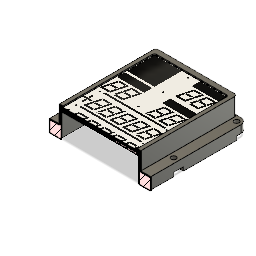
DSKY front frame mechanical 3D (Autodesk Fusion 360 design; units mm, degrees)
Autodesk Fusion 360 part; units mm, degrees
sketch "Sketch1" plane through (0, 0, 0) normal (0, 1, 0) x (1, 0, 0)
  line L0 (-36.322, 56.134) -> (36.322, 56.134)
  line L1 (41.402, 51.054) -> (41.402, -51.054)
  line L2 (36.322, -56.134) -> (-36.322, -56.134)
  line L3 (-41.402, -51.054) -> (-41.402, 51.054)
  line L4 (-41.402, 56.134) -> (41.402, -56.134) construction
  line L5 (41.402, 56.134) -> (-41.402, -56.134) construction
  arc A0 (-36.322, 56.134) -> (-41.402, 51.054) centre (-36.322, 51.054) ccw
  arc A1 (41.402, 51.054) -> (36.322, 56.134) centre (36.322, 51.054) ccw
  arc A2 (36.322, -56.134) -> (41.402, -51.054) centre (36.322, -51.054) ccw
  arc A3 (-41.402, -51.054) -> (-36.322, -56.134) centre (-36.322, -51.054) ccw
  line L6 (-30.988, 56.134) -> (30.988, 56.134)
  line L7 (33.274, 53.848) -> (33.274, -53.848)
  line L8 (30.988, -56.134) -> (-30.988, -56.134)
  line L9 (-33.274, -53.848) -> (-33.274, 53.848)
  line L10 (-33.274, 56.134) -> (33.274, -56.134) construction
  line L11 (33.274, 56.134) -> (-33.274, -56.134) construction
  arc A4 (-30.988, 56.134) -> (-33.274, 53.848) centre (-30.988, 53.848) ccw
  arc A5 (33.274, 53.848) -> (30.988, 56.134) centre (30.988, 53.848) ccw
  arc A6 (30.988, -56.134) -> (33.274, -53.848) centre (30.988, -53.848) ccw
  arc A7 (-33.274, -53.848) -> (-30.988, -56.134) centre (-30.988, -53.848) ccw
  line L12 (-28.702, 51.8795) -> (28.702, 51.8795)
  line L13 (30.226, 50.3555) -> (30.226, -50.3555)
  line L14 (28.702, -51.8795) -> (-28.702, -51.8795)
  line L15 (-30.226, -50.3555) -> (-30.226, 50.3555)
  line L16 (-30.226, 51.8795) -> (30.226, -51.8795) construction
  line L17 (30.226, 51.8795) -> (-30.226, -51.8795) construction
  arc A8 (-28.702, 51.8795) -> (-30.226, 50.3555) centre (-28.702, 50.3555) ccw
  arc A9 (30.226, 50.3555) -> (28.702, 51.8795) centre (28.702, 50.3555) ccw
  arc A10 (28.702, -51.8795) -> (30.226, -50.3555) centre (28.702, -50.3555) ccw
  arc A11 (-30.226, -50.3555) -> (-28.702, -51.8795) centre (-28.702, -50.3555) ccw
  line L18 (-30.456, 53.3795) -> (30.456, 53.3795)
  line L19 (31.726, 52.1095) -> (31.726, -52.1095)
  line L20 (30.456, -53.3795) -> (-30.456, -53.3795)
  line L21 (-31.726, -52.1095) -> (-31.726, 52.1095)
  line L22 (-31.726, 53.3795) -> (31.726, -53.3795) construction
  line L23 (31.726, 53.3795) -> (-31.726, -53.3795) construction
  arc A12 (-30.456, 53.3795) -> (-31.726, 52.1095) centre (-30.456, 52.1095) ccw
  arc A13 (31.726, 52.1095) -> (30.456, 53.3795) centre (30.456, 52.1095) ccw
  arc A14 (30.456, -53.3795) -> (31.726, -52.1095) centre (30.456, -52.1095) ccw
  arc A15 (-31.726, -52.1095) -> (-30.456, -53.3795) centre (-30.456, -52.1095) ccw
  line L24 (37.338, 51.562) -> (-37.338, 51.562) construction
  line L25 (-37.338, 51.562) -> (-37.338, -51.562) construction
  line L26 (-37.338, -51.562) -> (37.338, -51.562) construction
  line L27 (37.338, -51.562) -> (37.338, 51.562) construction
  line L28 (37.338, 51.562) -> (-37.338, -51.562) construction
  line L29 (-37.338, 51.562) -> (37.338, -51.562) construction
  circle A16 centre (-37.338, 51.562) radius 2.032
  circle A17 centre (37.338, 51.562) radius 2.032
  circle A18 centre (37.338, 0) radius 2.032
  circle A19 centre (37.338, -51.562) radius 2.032
  circle A20 centre (-37.338, -51.562) radius 2.032
  circle A21 centre (-37.338, 0) radius 2.032
  dimension "d1" = 82.804
  dimension "d2" = 112.268
  dimension "d3" = 5.08
  dimension "d4" = 66.548
  dimension "d5" = 2.286
  dimension "d6" = 60.452
  dimension "d7" = 103.759
  dimension "d8" = 1.524
  dimension "d15" = 1.5
  dimension "d16" = 1.5
  dimension "d17" = 1.27
  dimension "d21" = 4.064
  dimension "d22" = 74.676
  dimension "d23" = 103.124
  measures "d3" radius of A0
  measures "d4" distance of L7 L9
  measures "d5" radius of A4
  measures "d8" radius of A8
  measures "d15" distance of L12 L18
  measures "d16" distance of L15 L21
  measures "d17" radius of A12
  measures "d21" diameter of A17
  measures "d22" distance of L25 L27
  measures "d23" distance of L24 L26
extrude "Extrude1" add sketch "Sketch1" against normal blind 23.876 contours L0 L2 L3 A0 A3 L9 A4 A7 | L0 L2 L6 L7 L8 L9 A4 A5 A6 A7 | L0 L1 L2 A1 A2 L7 A5 A6 | L12 L13 L14 L15 A8 A9 A10 A11 | L18 L19 L20 L21 A12 A13 A14 A15 | A16 | A17 | A18 | A19 | A20 | A21 makes body 1
extrude "Extrude2" cut sketch "Sketch1" against normal blind 14.351 contours L0 L2 L3 A0 A3 L9 A4 A7 | L0 L1 L2 A1 A2 L7 A5 A6 | A16 | A17 | A18 | A19 | A20 | A21 bodies 1
extrude "Extrude3" cut sketch "Sketch1" against normal blind 70 contours L12 L13 L14 L15 A8 A9 A10 A11 bodies 1
extrude "Extrude4" cut sketch "Sketch1" against normal blind 40 from surface at -1 contours L18 L19 L20 L21 A12 A13 A14 A15 bodies 1
extrude "Extrude5" cut sketch "Sketch1" against normal blind 80 contours A16 | A17 | A18 | A19 | A20 | A21 bodies 1
sketch "Sketch2" plane through (0, -23.876, 0) normal (0, -1, 0) x (1, 0, 0)
  circle A0 centre (37.338, 51.562) radius 2.032
  circle A1 centre (-37.338, -51.562) radius 2.032
  circle A2 centre (37.338, 0) radius 2.032
  circle A3 centre (-37.338, 51.562) radius 2.032
  circle A4 centre (-37.338, 0) radius 2.032
  circle A5 centre (37.338, -51.562) radius 2.032
  line L0 (-31.726, -52.1095) -> (-31.726, 52.1095)
  arc A6 (-30.456, 53.3795) -> (-31.726, 52.1095) centre (-30.456, 52.1095) ccw
  line L1 (-30.456, 53.3795) -> (30.456, 53.3795)
  arc A7 (31.726, 52.1095) -> (30.456, 53.3795) centre (30.456, 52.1095) ccw
  line L2 (31.726, 52.1095) -> (31.726, -52.1095)
  arc A8 (30.456, -53.3795) -> (31.726, -52.1095) centre (30.456, -52.1095) ccw
  line L3 (30.456, -53.3795) -> (-30.456, -53.3795)
  arc A9 (-31.726, -52.1095) -> (-30.456, -53.3795) centre (-30.456, -52.1095) ccw
  arc A10 (41.402, 51.054) -> (36.322, 56.134) centre (36.322, 51.054) ccw
  line L4 (36.322, 56.134) -> (-36.322, 56.134)
  arc A11 (-36.322, 56.134) -> (-41.402, 51.054) centre (-36.322, 51.054) ccw
  line L5 (-41.402, 51.054) -> (-41.402, -51.054)
  arc A12 (-41.402, -51.054) -> (-36.322, -56.134) centre (-36.322, -51.054) ccw
  line L6 (-36.322, -56.134) -> (36.322, -56.134)
  arc A13 (36.322, -56.134) -> (41.402, -51.054) centre (36.322, -51.054) ccw
  line L7 (41.402, -51.054) -> (41.402, 51.054)
  line L8 (-33.528, 51.562) -> (-33.528, 57.6053)
  line L9 (-33.528, 57.6053) -> (-43.8706, 57.6053)
  line L10 (-37.338, 47.752) -> (-43.8706, 47.752)
  line L11 (-43.8706, 47.752) -> (-43.8706, 57.6053)
  arc A14 (-37.338, 47.752) -> (-33.528, 51.562) centre (-37.338, 51.562) ccw
  line L12 (-37.338, 3.81) -> (-44.0815, 3.81)
  line L13 (-44.0815, 3.81) -> (-44.0815, -3.81)
  line L14 (-37.338, -3.81) -> (-44.0815, -3.81)
  arc A15 (-37.338, -3.81) -> (-37.338, 3.81) centre (-37.338, 0) ccw
  line L15 (-37.338, -47.752) -> (-43.7202, -47.752)
  line L16 (-43.7202, -47.752) -> (-43.7202, -57.2057)
  line L17 (-33.528, -51.562) -> (-33.528, -57.2057)
  line L18 (-33.528, -57.2057) -> (-43.7202, -57.2057)
  arc A16 (-33.528, -51.562) -> (-37.338, -47.752) centre (-37.338, -51.562) ccw
  line L19 (0, 0) -> (0, 74.1902) construction
  line L20 (33.528, 57.6053) -> (43.8706, 57.6053)
  line L21 (43.8706, 47.752) -> (43.8706, 57.6053)
  line L22 (37.338, 47.752) -> (43.8706, 47.752)
  arc A17 (33.528, 51.562) -> (37.338, 47.752) centre (37.338, 51.562) ccw
  line L23 (33.528, 51.562) -> (33.528, 57.6053)
  arc A18 (37.338, 3.81) -> (37.338, -3.81) centre (37.338, 0) ccw
  line L24 (37.338, 3.81) -> (44.0815, 3.81)
  line L25 (44.0815, 3.81) -> (44.0815, -3.81)
  line L26 (37.338, -3.81) -> (44.0815, -3.81)
  line L27 (43.7202, -47.752) -> (43.7202, -57.2057)
  line L28 (33.528, -57.2057) -> (43.7202, -57.2057)
  line L29 (33.528, -51.562) -> (33.528, -57.2057)
  arc A19 (37.338, -47.752) -> (33.528, -51.562) centre (37.338, -51.562) ccw
  line L30 (37.338, -47.752) -> (43.7202, -47.752)
  dimension "d26" = 3.81
  measures "d26" radius of A14
extrude "Extrude6" cut sketch "Sketch2" against normal blind 3.175 contours A10 L4 L7 L22 A17 L23 | L7 A18 L24 L26 | L4 A11 L5 L8 L10 A14 | L6 A13 L7 L29 A19 L30 | L5 L12 L14 A15 | L5 A12 L6 L15 L17 A16 bodies 1
sketch "Sketch3" plane through (0, -1, 0) normal (0, -1, 0) x (1, 0, 0)
  arc A0 (-30.226, -50.3555) -> (-28.702, -51.8795) centre (-28.702, -50.3555) ccw
  line L0 (-30.226, -50.3555) -> (-30.226, 50.3555)
  arc A1 (-28.702, 51.8795) -> (-30.226, 50.3555) centre (-28.702, 50.3555) ccw
  line L1 (-28.702, 51.8795) -> (28.702, 51.8795)
  arc A2 (30.226, 50.3555) -> (28.702, 51.8795) centre (28.702, 50.3555) ccw
  line L2 (30.226, 50.3555) -> (30.226, -50.3555)
  arc A3 (28.702, -51.8795) -> (30.226, -50.3555) centre (28.702, -50.3555) ccw
  line L3 (28.702, -51.8795) -> (-28.702, -51.8795)
  arc A4 (-31.726, -52.1095) -> (-30.456, -53.3795) centre (-30.456, -52.1095) ccw
  line L4 (-30.456, -53.3795) -> (30.456, -53.3795)
  arc A5 (30.456, -53.3795) -> (31.726, -52.1095) centre (30.456, -52.1095) ccw
  line L5 (31.726, -52.1095) -> (31.726, 52.1095)
  arc A6 (31.726, 52.1095) -> (30.456, 53.3795) centre (30.456, 52.1095) ccw
  line L6 (30.456, 53.3795) -> (-30.456, 53.3795)
  arc A7 (-30.456, 53.3795) -> (-31.726, 52.1095) centre (-30.456, 52.1095) ccw
  line L7 (-31.726, 52.1095) -> (-31.726, -52.1095)
  arc A8 (-31.218, -52.1095) -> (-30.456, -52.8715) centre (-30.456, -52.1095) ccw
  line L8 (-30.456, -52.8715) -> (30.456, -52.8715)
  arc A9 (30.456, -52.8715) -> (31.218, -52.1095) centre (30.456, -52.1095) ccw
  line L9 (31.218, -52.1095) -> (31.218, 52.1095)
  arc A10 (31.218, 52.1095) -> (30.456, 52.8715) centre (30.456, 52.1095) ccw
  line L10 (30.456, 52.8715) -> (-30.456, 52.8715)
  arc A11 (-30.456, 52.8715) -> (-31.218, 52.1095) centre (-30.456, 52.1095) ccw
  line L11 (-31.218, 52.1095) -> (-31.218, -52.1095)
  dimension "d29" = 0.508
extrude "Extrude7" add sketch "Sketch3" along normal blind 1.1 separate body contours A0 L0 A1 L1 A2 L2 A3 L3 | A8 L8 A9 L9 A10 L10 A11 L11 makes body 2
sketch "Sketch4" plane through (0, -2.1, 0) normal (0, -1, 0) x (1, 0, 0)
  line L0 (-31.218, 52.1095) -> (-31.218, -52.1095)
  arc A0 (-31.218, -52.1095) -> (-30.456, -52.8715) centre (-30.456, -52.1095) ccw
  line L1 (-30.456, -52.8715) -> (30.456, -52.8715)
  arc A1 (30.456, -52.8715) -> (31.218, -52.1095) centre (30.456, -52.1095) ccw
  line L2 (31.218, -52.1095) -> (31.218, 52.1095)
  arc A2 (31.218, 52.1095) -> (30.456, 52.8715) centre (30.456, 52.1095) ccw
  line L3 (30.456, 52.8715) -> (-30.456, 52.8715)
  arc A3 (-30.456, 52.8715) -> (-31.218, 52.1095) centre (-30.456, 52.1095) ccw
  line L4 (-30.456, -52.8715) -> (30.456, -52.8715)
  arc A4 (30.456, -52.8715) -> (31.218, -52.1095) centre (30.456, -52.1095) ccw
  line L5 (31.218, -52.1095) -> (31.218, 52.1095)
  arc A5 (31.218, 52.1095) -> (30.456, 52.8715) centre (30.456, 52.1095) ccw
  line L6 (30.456, 52.8715) -> (-30.456, 52.8715)
  arc A6 (-30.456, 52.8715) -> (-31.218, 52.1095) centre (-30.456, 52.1095) ccw
  line L7 (-31.218, 52.1095) -> (-31.218, -52.1095)
  arc A7 (-31.218, -52.1095) -> (-30.456, -52.8715) centre (-30.456, -52.1095) ccw
  dimension "d32" = 0
  measures "d32" distance of L1
extrude "Extrude8" add sketch "Sketch4" along normal blind 1.524 from surface at 0.127 separate body makes body 3
